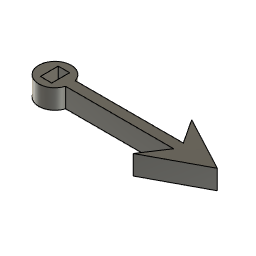
Flecha_motor_a_pasos_28BYJ-48 (Autodesk Fusion 360 design; units mm, degrees)
Autodesk Fusion 360 part; units mm, degrees
sketch "Sketch1" plane through (0, 0, 0) normal (0, 0, 1) x (1, 0, 0)
  line L0 (38.058, -1.5) -> (4.7697, -1.5)
  line L1 (4.7697, 1.5) -> (38.0528, 1.5)
  line L2 (50, 0) -> (33.1127, 8.996)
  line L3 (33.1127, -9.004) -> (50, 0)
  line L4 (33.1127, -9.004) -> (38.058, -1.5)
  line L5 (38.0528, 1.5) -> (33.1127, 8.996)
  arc A0 (4.7697, 1.5) -> (4.7697, -1.5) centre (0, 0) ccw
  point P0 (33.1127, 8.996)
  point P1 (33.1127, -9.004)
  point P2 (39.044, -0.004)
  dimension "d1" = 10
  constraint horizontal L0
  constraint parallel L0 L1
  constraint coincident P0 L2.end
  constraint coincident P1 L3.start
  measures "d1" diameter of A0
extrude "Extrude1" add sketch "Sketch1" along normal blind 6
sketch "Sketch2" plane through (0, 0, 6) normal (0, 0, 1) x (-1, 0, 0)
  line L0 (-38.0528, -1.5) -> (-4.7697, -1.5)
  arc A0 (-4.7697, -1.5) -> (-4.7697, 1.5) centre (0, 0) ccw
  line L1 (-4.7697, 1.5) -> (-38.058, 1.5)
  line L2 (-38.058, 1.5) -> (-33.1127, 9.004)
  line L3 (-33.1127, 9.004) -> (-50, 0)
  line L4 (-50, 0) -> (-33.1127, -8.996)
  line L5 (-33.1127, -8.996) -> (-38.0528, -1.5)
  line L6 (1.75, -2.75) -> (-1.75, -2.75)
  line L7 (-1.75, -2.75) -> (-1.75, 2.75)
  line L8 (-1.75, 2.75) -> (1.75, 2.75)
  line L9 (1.75, 2.75) -> (1.75, -2.75)
  line L10 (1.75, -2.75) -> (-1.75, 2.75) construction
  line L11 (-1.75, -2.75) -> (1.75, 2.75) construction
  dimension "d9" = 3.5
  dimension "d10" = 5.5
  constraint horizontal L6
  constraint perpendicular L6 L7
  constraint parallel L6 L8
  constraint parallel L7 L9
  constraint coincident L10 A0.centre
  constraint coincident L11 A0.centre
  constraint coincident A0.centre origin
  measures "d9" distance of L7.end L8.end
  measures "d10" distance of L6.start L8.end
extrude "Extrude2" cut sketch "Sketch2" against normal blind 6 contours L6 L7 L8 L9
